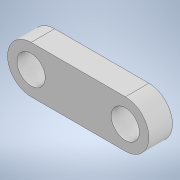
# Autodesk Inventor part: Part5
Saved by Autodesk Inventor 2022 (Build 260153000, 153)
## iProperties
Created: 2022-02-01
Part Number: Part5
Material: Generic
Document SubType Name: Modeling
Designer: br4ch
Density: 1 g/cm^3
Appearance: Default
Author: br4ch
Autodesk Inventor part; units mm, degrees
ref_plane "YZ Plane" through (0, 0, 0) normal (1, 0, 0) x (0, 1, 0)
ref_plane "XZ Plane" through (0, 0, 0) normal (0, 1, 0) x (-1, 0, 0)
ref_plane "XY Plane" through (0, 0, 0) normal (0, 0, 1) x (1, 0, 0)
sketch "Sketch1" plane through (0, 0, 0) normal (0, 0, 1) x (1, 0, 0)
  line L0 (-37.3186, 10.7459) -> (-17.3186, 10.7459) construction
  line L1 (-37.3186, 5.7459) -> (-17.3186, 5.7459)
  line L2 (-17.3186, 15.7459) -> (-37.3186, 15.7459)
  arc A0 (-37.3186, 15.7459) -> (-37.3186, 5.7459) centre (-37.3186, 10.7459) ccw
  arc A1 (-17.3186, 5.7459) -> (-17.3186, 15.7459) centre (-17.3186, 10.7459) ccw
  circle A2 centre (-37.3186, 10.7459) radius 3
  circle A3 centre (-17.3186, 10.7459) radius 3
  point P0 (0, 0)
  point P1 (-27.3186, 10.7459)
  dimension "d0" = 10
  dimension "d5" = 20
  dimension "d6" = 6
  constraints: 8 end point, 4 centre point, 4 point on circle, 4 tangent, 2 coincident, 1 equal radius, 1 horizontal, 1 midpoint, 1 parallel
  measures "d0" diameter of A1
  measures "d5" distance of L0.end L0.start
  measures "d6" diameter of A2
extrude "Extrusion1" add sketch "Sketch1" along normal blind 5
equation "\"d0\" = R"
equation "\"d6\" = r"
equation "\"d3\" = th"
equation "\"th\" = 5"
equation "\"r\" = 6"
equation "\"R\" = 10"
body "Solid1"
